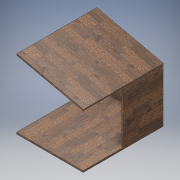
# Autodesk Inventor part: Top
Saved by Autodesk Inventor 2017 (Build 210142000, 142)
## iProperties
Created: 2016-09-09
Part Number: Top
Material: Generic
Document SubType Name: Modeling
Designer: s.ethan.wierenga
Density: 1 g/cm^3
Appearance: White Ash - Java
Author: s.ethan.wierenga
Autodesk Inventor part; units mm, degrees
ref_plane "YZ Plane" through (0, 0, 0) normal (1, 0, 0) x (0, 1, 0)
ref_plane "XZ Plane" through (0, 0, 0) normal (0, 1, 0) x (-1, 0, 0)
ref_plane "XY Plane" through (0, 0, 0) normal (0, 0, 1) x (1, 0, 0)
sketch "Sketch1" plane through (0, 0, 0) normal (0, 1, 0) x (-1, 0, 0)
  line L0 (0, 0) -> (-762, 0)
  line L1 (-762, 0) -> (-762, -914.4)
  line L2 (-762, -914.4) -> (0, -914.4)
  line L3 (0, -914.4) -> (0, 0)
  dimension "d0" = 762
  dimension "d1" = 914.4
  constraints: 8 end point, 2 parallel, 1 horizontal, 1 perpendicular
  measures "d0" distance of L2.end L1.end
  measures "d1" distance of L1.end L0.end
extrude "Extrusion1" add sketch "Sketch1" along normal blind 19.05
sketch "Sketch5" plane through (762, 0, -914.4) normal (0, 0, -1) x (-1, 0, 0)
  line L0 (0, 0) -> (0, 19.05) projected
  line L1 (0, 0) -> (762, 0) projected
  line L2 (762, 0) -> (762, 19.05) projected
  line L3 (762, 628.65) -> (762, 781.05)
  line L4 (762, 781.05) -> (0, 609.6)
  line L5 (0, 609.6) -> (762, 609.6) construction
  line L6 (762, 19.05) -> (762, 628.65) construction
  line L7 (762, 781.05) -> (757.8183, 799.6354)
  line L8 (757.8183, 799.6354) -> (-4.1817, 628.1854)
  line L9 (0, 609.6) -> (84.6693, 628.65) projected
  line L10 (-4.1817, 628.1854) -> (0, 609.6)
  line L11 (0, 19.05) -> (762, 19.05) projected
  dimension "d22" = 152.4
  dimension "d23" = 12.68
  dimension "d25" = 19.05
  dimension "d26" = 90
  dimension "d28" = 90
  dimension "d29" = 90
  constraints: 12 end point, 1 perpendicular, 1 point on line, 1 vertical
  measures "d22" distance of L3.start L3.end
  measures "d23" angle of L5 L4
  measures "d25" distance of L3.end L7.end
  measures "d26" angle of L7 L4
  measures "d28" angle of L4 L10
  measures "d29" angle of L8 L10
extrude "Extrusion5" add sketch "Sketch5" against normal up to surface (914.4 mm away) contours L4 L10 L8 L7
sketch "Sketch7" plane through (0, 19.05, 0) normal (0, 1, 0) x (1, 0, 0)
  line L0 (0, 0) -> (762, 0) projected
  line L1 (0, 914.4) -> (0, 0) projected
  line L2 (762, 914.4) -> (0, 914.4) projected
  line L3 (762, 0) -> (762, 914.4) projected
  line L4 (762, 0) -> (762, 914.4) projected
  line L5 (0, 914.4) -> (0, 0) projected
  line L6 (762, 914.4) -> (0, 914.4)
  line L7 (0, 914.4) -> (0, 895.35)
  line L8 (0, 895.35) -> (742.95, 895.35)
  line L9 (762, 895.35) -> (762, 914.4)
  line L10 (762, 914.4) -> (742.95, 914.4)
  line L11 (742.95, 895.35) -> (742.95, 457.2)
  line L12 (742.95, 457.2) -> (762, 457.2)
  line L13 (762, 457.2) -> (762, 914.4)
  dimension "d38" = 19.05
  dimension "d39" = 19.05
  dimension "d40" = 457.2
  constraints: 16 end point, 4 parallel, 2 horizontal, 2 perpendicular, 1 point on line
  measures "d38" distance of L7.end L6.end
  measures "d39" distance of L12.end L11.end
  measures "d40" distance of L11.end L10.end
extrude "Extrusion7" add sketch "Sketch7" along normal blind 609.6 contours L1 L2 L3 L12 L11 L8
sketch "Sketch8" plane through (762, 0, -914.4) normal (0, 0, -1) x (-1, 0, 0)
  line L0 (0, 0) -> (762, 0) projected
  line L1 (762, 0) -> (762, 628.65) projected
  line L2 (84.6667, 628.65) -> (762, 628.65) projected
  line L3 (84.6667, 628.65) -> (762, 781.05) projected
  line L4 (762, 781.05) -> (757.8183, 799.6354) projected
  line L5 (757.8183, 799.6354) -> (-4.1817, 628.1854) projected
  line L6 (-4.1817, 628.1854) -> (0, 609.6) projected
  line L7 (0, 0) -> (0, 609.6) projected
  line L8 (762, 628.65) -> (762, 781.05)
  line L9 (84.6667, 628.65) -> (762, 781.05) projected
  line L10 (762, 781.05) -> (84.6667, 628.65)
  line L11 (84.6667, 628.65) -> (762, 628.65)
  constraints: 6 end point, 1 collinear, 1 perpendicular, 1 vertical
extrude "Extrusion8" add sketch "Sketch8" against normal blind 19.05 contours L2 L3 L8
body "Solid1"
